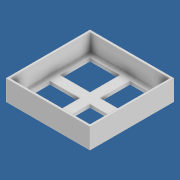
# Autodesk Inventor part: test plate
Saved by Autodesk Inventor 2020 (Build 240168000, 168)
## iProperties
Created: 2021-09-04
Part Number: test plate
Material: Generic
Document SubType Name: Modeling
Designer: RNG3nius
Density: 1 g/cm^3
Appearance: Default
Author: RNG3nius
Autodesk Inventor part; units mm, degrees
ref_plane "YZ Plane" through (0, 0, 0) normal (1, 0, 0) x (0, 1, 0)
ref_plane "XZ Plane" through (0, 0, 0) normal (0, 1, 0) x (-1, 0, 0)
ref_plane "XY Plane" through (0, 0, 0) normal (0, 0, 1) x (1, 0, 0)
sketch "Sketch1" plane through (0, 0, 0) normal (0, 1, 0) x (-1, 0, 0)
  line L0 (0, 0) -> (41.3, 0)
  line L1 (41.3, 0) -> (41.3, 41.3)
  line L2 (41.3, 41.3) -> (0, 41.3)
  line L3 (0, 41.3) -> (0, 0)
  dimension "d0" = 41.3
  dimension "d1" = 41.3
  constraints: 8 end point, 2 parallel, 1 horizontal, 1 perpendicular
  measures "d0" distance of L2.end L1.end
  measures "d1" distance of L1.end L0.end
extrude "Extrusion1" add sketch "Sketch1" along normal blind 10
sketch "Sketch8" plane through (0, 10, 0) normal (0, 1, 0) x (1, 0, 0)
  line L0 (-1, -1) -> (-40.3, -1)
  line L1 (-40.3, -1) -> (-40.3, -40.3)
  line L2 (-40.3, -40.3) -> (-1, -40.3)
  line L3 (-1, -40.3) -> (-1, -1)
  line L4 (0, 0) -> (-41.3, 0) projected
  line L5 (0, -41.3) -> (0, 0) projected
  dimension "d61" = 39.3
  dimension "d62" = 39.3
  dimension "d63" = 1
  dimension "d64" = 1
  constraints: 8 end point, 2 parallel, 1 horizontal, 1 perpendicular
  measures "d61" distance of L2.end L1.end
  measures "d62" distance of L1.end L0.end
  measures "d63" distance between parallel lines of L4 L0
  measures "d64" distance between parallel lines of L5 L3
extrude "Extrusion7" cut sketch "Sketch8" against normal blind 8.5
sketch "Sketch9" plane through (0, 1.5, 0) normal (0, 1, 0) x (1, 0, 0)
  line L0 (-3.45, -3.45) -> (-18.15, -3.45)
  line L1 (-18.15, -3.45) -> (-18.15, -18.15)
  line L2 (-18.15, -18.15) -> (-3.45, -18.15)
  line L3 (-3.45, -18.15) -> (-3.45, -3.45)
  line L4 (-1, -1) -> (-1, -40.3) projected
  line L5 (-40.3, -1) -> (-1, -1) projected
  line L6 (-23.15, -3.45) -> (-37.85, -3.45)
  line L7 (-37.85, -3.45) -> (-37.85, -18.15)
  line L8 (-37.85, -18.15) -> (-23.15, -18.15)
  line L9 (-23.15, -18.15) -> (-23.15, -3.45)
  line L10 (-23.15, -23.15) -> (-37.85, -23.15)
  line L11 (-37.85, -23.15) -> (-37.85, -37.85)
  line L12 (-37.85, -37.85) -> (-23.15, -37.85)
  line L13 (-23.15, -37.85) -> (-23.15, -23.15)
  line L14 (-40.3, -40.3) -> (-40.3, -1) projected
  line L15 (-18.15, -23.15) -> (-3.45, -23.15)
  line L16 (-3.45, -23.15) -> (-3.45, -37.85)
  line L17 (-3.45, -37.85) -> (-18.15, -37.85)
  line L18 (-18.15, -37.85) -> (-18.15, -23.15)
  point P0 (0, 0)
  dimension "d67" = 14.7
  dimension "d68" = 14.7
  dimension "d69" = 2.45
  dimension "d70" = 2.45
  dimension "d71" = 14.7
  dimension "d72" = 14.7
  dimension "d73" = 5
  dimension "d74" = 14.7
  dimension "d75" = 14.7
  dimension "d76" = 5
  dimension "d77" = 2.45
  dimension "d78" = 14.7
  dimension "d79" = 14.7
  dimension "d80" = 5
  dimension "d81" = 5
  constraints: 32 end point, 8 parallel, 4 horizontal, 4 perpendicular, 1 point on line
  measures "d67" distance of L2.end L1.end
  measures "d68" distance of L1.end L0.end
  measures "d69" distance between parallel lines of L3 L4
  measures "d70" distance between parallel lines of L5 L0
  measures "d71" distance of L8.end L7.end
  measures "d72" distance of L7.end L6.end
  measures "d73" distance between parallel lines of L9 L1
  measures "d74" distance of L12.end L11.end
  measures "d75" distance of L11.end L10.end
  measures "d76" distance between parallel lines of L8 L10
  measures "d77" distance between parallel lines of L14 L11
  measures "d78" distance of L16.end L17.end
  measures "d79" distance of L15.end L16.end
  measures "d80" distance between parallel lines of L13 L18
  measures "d81" distance between parallel lines of L2 L15
extrude "Extrusion8" cut sketch "Sketch9" against normal blind 8.5
body "Solid1"
